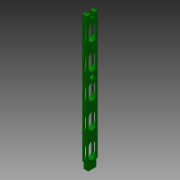
# Autodesk Inventor part: 13_1087_003
Saved by Autodesk Inventor 2014 (Build 180170000, 170)
## iProperties
Created: 2013-08-01
Part Number: 13_1087_003
Material: Bronze (weiche Zinnbronze)
Document SubType Name: Modeling
Designer: vogel
Density: 8.874 g/cm^3
Appearance: Dunkelgrün
Author: vogel
Autodesk Inventor part; units mm, degrees
note: some values were not read from the file. Chosen so that the rebuilt part matches the saved one: direction of "Bohrung6"; direction of "Bohrung8".
ref_plane "YZ Plane" through (0, 0, 0) normal (1, 0, 0) x (0, 1, 0)
ref_plane "XZ Plane" through (0, 0, 0) normal (0, 1, 0) x (-1, 0, 0)
ref_plane "XY Plane" through (0, 0, 0) normal (0, 0, 1) x (1, 0, 0)
sketch "Skizze1" plane through (0, 0, 0) normal (0, 0, 1) x (1, 0, 0)
  line L0 (-3.5, 0) -> (3.5, 0) projected
  line L1 (0, -8.4) -> (0, 8.4) projected
  line L2 (-2.5, 6) -> (2.5, 6)
  line L3 (2.5, 6) -> (2.5, -6)
  line L4 (2.5, -6) -> (-2.5, -6)
  line L5 (-2.5, -6) -> (-2.5, 6)
  point P0 (0, 0)
  dimension "d0" = 12
  dimension "d1" = 5
  constraints: 8 end point, 2 parallel, 1 horizontal, 1 perpendicular, 2 other
  measures "d0" distance between parallel lines of L4 L2
  measures "d1" distance of L2.start L2.end
extrude "Extrusion1" add sketch "Skizze1" along normal blind 150
sketch "Skizze2" plane through (2.5, -6, 0) normal (1, 0, 0) x (0, 0, -1)
  line L0 (0, -2.4) -> (0, 14.4) projected
  line L1 (30, 6) -> (-180, 6) projected
  line L2 (-8, 10.5) -> (0, 10.5)
  line L3 (0, 10.5) -> (0, 12)
  line L4 (0, 12) -> (-8, 12)
  line L5 (-8, 12) -> (-8, 10.5)
  line L6 (0, 0) -> (-8, 0)
  line L7 (-8, 0) -> (-8, 1.5)
  line L8 (-8, 1.5) -> (0, 1.5)
  line L9 (0, 1.5) -> (0, 0)
  point P0 (0, 6)
  dimension "d4" = 8
  dimension "d5" = 9
  constraints: 16 end point, 4 parallel, 2 horizontal, 2 perpendicular, 1 collinear, 1 other
  measures "d4" distance of L7.end L8.end
  measures "d5" distance between parallel lines of L8 L2
extrude "Extrusion2" cut sketch "Skizze2" against normal through all
sketch "Skizze3" plane through (0, 0, 150) normal (0, 0, 1) x (1, 0, 0)
  line L0 (-2.5, 6) -> (-2.5, -6) projected
  line L1 (-2.5, 2.5) -> (1.5, 2.5)
  line L2 (1.5, 2.5) -> (1.5, -2.5)
  line L3 (1.5, -2.5) -> (-2.5, -2.5)
  line L4 (-2.5, -2.5) -> (-2.5, 2.5)
  line L5 (-3.5, 0) -> (3.5, 0) projected
  line L6 (0, -8.4) -> (0, 8.4) projected
  point P0 (0, 0)
  dimension "d8" = 5
  dimension "d9" = 4
  constraints: 8 end point, 2 parallel, 1 horizontal, 1 perpendicular, 1 point on line, 1 other
  measures "d8" distance between parallel lines of L3 L1
  measures "d9" distance between parallel lines of L0 L2
extrude "Extrusion3" cut sketch "Skizze3" against normal blind 15
fillet "Rundung1" radius 2.5 2 edges at (-0.5, 2.5, 135) (-0.5, -2.5, 135)
sketch "Skizze4" plane through (-2.5, -6, 150) normal (0, -1, 0) x (1, 0, 0)
  line L0 (0, 0) -> (5, 0) projected
  line L1 (0, -142) -> (0, 0) projected
  line L2 (2, 0) -> (2, -7.1853)
  point P0 (2.5, -150)
  point P1 (2, -2)
  dimension "d13" = 2
  dimension "d14" = 2
  constraints: 2 end point, 2 point on line, 1 parallel
  measures "d13" distance from line of point (2, -2) L0
  measures "d14" distance between parallel lines of L1 L2
hole "Bohrung1" at (-0.5, -6, 148) direction (0, 1, 0) diameter 2 end through all
sketch "Skizze5" plane through (2.5, -6, 150) normal (1, 0, 0) x (0, 0, -1)
  line L0 (0, 0) -> (0, 12) projected
  line L1 (0, 8.5) -> (4, 8.5)
  line L2 (4, 8.5) -> (4, 3.5)
  line L3 (4, 3.5) -> (0, 3.5)
  line L4 (0, 3.5) -> (0, 8.5)
  line L5 (150, -2.4) -> (150, 14.4) projected
  line L6 (180, 6) -> (-30, 6) projected
  point P0 (150, 6)
  dimension "d22" = 5
  dimension "d23" = 4
  constraints: 8 end point, 2 parallel, 1 horizontal, 1 perpendicular, 1 point on line, 1 other
  measures "d22" distance between parallel lines of L3 L1
  measures "d23" distance between parallel lines of L0 L2
extrude "Extrusion4" cut sketch "Skizze5" against normal through all
sketch "Skizze6" plane through (0, 0, 0) normal (0, 0, -1) x (-1, 0, 0)
  point P0 (0, 0)
  point P1 (0, 0)
  constraints: 1 coincident
hole "Bohrung2" at (0, 0, 0) direction (0, 0, 1) diameter 1.567 depth 6 tip angle 118 thread size "M2x0.4" class "6H" standard "ISO Metric profile"
sketch "Skizze10" plane through (-2.5, 6, 150) normal (0, 1, 0) x (1, 0, 0)
  line L0 (5, 142) -> (0, 142) projected
  line L1 (5, 142) -> (5, 0) projected
  line L2 (2.5, 137) -> (2.5, 127) construction
  line L3 (1, 137) -> (1, 127)
  line L4 (4, 127) -> (4, 137)
  arc A0 (4, 137) -> (1, 137) centre (2.5, 137) ccw
  arc A1 (1, 127) -> (4, 127) centre (2.5, 127) ccw
  point P0 (2.5, 150)
  point P1 (2.5, 132)
  dimension "d63" = 5
  dimension "d64" = 2.5
  dimension "d65" = 3
  dimension "d66" = 10
  constraints: 8 end point, 4 point on circle, 4 tangent, 2 centre point, 2 parallel, 1 midpoint
  measures "d63" distance from line of L2.start L0
  measures "d64" distance between parallel lines of L2 L1
  measures "d65" distance between parallel lines of L3 L4
  measures "d66" distance of L2.end L2.start
extrude "Extrusion5" cut sketch "Skizze10" against normal through all
pattern_linear "Rechteckige Anordnung2" count 5 spacing 28.4 along (0, 0, 1) of "Extrusion5"
sketch "Skizze11" plane through (2.5, -4.5, 0) normal (1, 0, 0) x (0, 0, -1)
  line L0 (-8, -1.5) -> (-150, -1.5) projected
  line L1 (-8, -1.5) -> (-8, 0) projected
  line L2 (-13, 4.5) -> (-23, 4.5) construction
  line L3 (-13, 0.5) -> (-23, 0.5)
  line L4 (-23, 8.5) -> (-13, 8.5)
  arc A0 (-13, 0.5) -> (-13, 8.5) centre (-13, 4.5) ccw
  arc A1 (-23, 8.5) -> (-23, 0.5) centre (-23, 4.5) ccw
  point P0 (0, 4.5)
  point P1 (-18, 4.5)
  dimension "d72" = 5
  dimension "d73" = 8
  dimension "d74" = 6
  dimension "d75" = 10
  constraints: 8 end point, 4 point on circle, 4 tangent, 2 centre point, 2 parallel, 1 midpoint
  measures "d72" distance from line of L2.start L1
  measures "d73" distance between parallel lines of L4 L3
  measures "d74" distance between parallel lines of L2 L0
  measures "d75" distance of L2.end L2.start
extrude "Extrusion6" cut sketch "Skizze11" against normal through all
pattern_linear "Rechteckige Anordnung3" count 5 spacing 28.4 along (0, 0, 1) of "Extrusion6"
sketch "Skizze12" plane through (-2.5, 6, 150) normal (0, 1, 0) x (1, 0, 0)
  line L0 (0, 142) -> (0, 0) projected
  line L1 (5, 0) -> (0, 0) projected
  line L2 (5, 142) -> (5, 0) projected
  line L3 (2, 0) -> (2, 6.9396)
  point P0 (2.5, 150)
  point P1 (2, 8)
  dimension "d81" = 2
  dimension "d82" = 8
  constraints: 2 end point, 2 point on line, 1 parallel
  measures "d81" distance between parallel lines of L0 L3
  measures "d82" distance from line of point (2, 8) L1
hole "Bohrung6" at (-0.5, 6, 142) direction (0, -1, 0) diameter 2.459 end up to surface thread size "M3x0.5" class "6H" standard "ISO Metric profile"
sketch "Skizze13" plane through (2.5, -4.5, 0) normal (1, 0, 0) x (0, 0, -1)
  arc A0 (-98.2, 0.5) -> (-98.2, 8.5) centre (-98.2, 4.5) ccw projected
  arc A1 (-79.8, 8.5) -> (-79.8, 0.5) centre (-79.8, 4.5) ccw projected
  line L0 (-8, -1.5) -> (-150, -1.5) projected
  line L1 (-8, 10.5) -> (-150, 10.5) projected
  line L2 (-150, 7) -> (-150, 10.5) projected
  line L3 (-98.2, 4.5) -> (-79.8, 4.5)
  line L4 (-89, 10.5) -> (-89, -1.5)
  point P0 (0, 4.5)
  point P1 (-89, 4.5)
  constraints: 4 end point, 2 coincident, 2 perpendicular, 2 point on line, 1 midpoint, 1 symmetric about line
hole "Bohrung7" at (2.5, 0, 98.2) at (2.5, 0, 79.8) at (2.5, 0, 89) direction (-1, 0, 0) diameter 5 end through all
sketch "Skizze14" plane through (-2.5, 6, 150) normal (0, 1, 0) x (1, 0, 0)
  arc A0 (4, 51.8) -> (1, 51.8) centre (2.5, 51.8) ccw projected
  arc A1 (1, 70.2) -> (4, 70.2) centre (2.5, 70.2) ccw projected
  line L0 (5, 142) -> (5, 0) projected
  line L1 (2.5, 70.2) -> (2.5, 51.8)
  line L2 (1, 61) -> (4, 61)
  line L3 (1.75, 51.8) -> (2.5, 51.8)
  line L4 (2.5, 70.2) -> (1.75, 70.2)
  point P0 (2.5, 150)
  point P1 (2.5, 61)
  constraints: 8 end point, 3 parallel, 2 midpoint, 1 perpendicular, 1 other
hole "Bohrung8" at (0, 6, 89) direction (0, -1, 0) diameter 2.459 end up to surface thread size "M3x0.5" class "6H" standard "ISO Metric profile"
